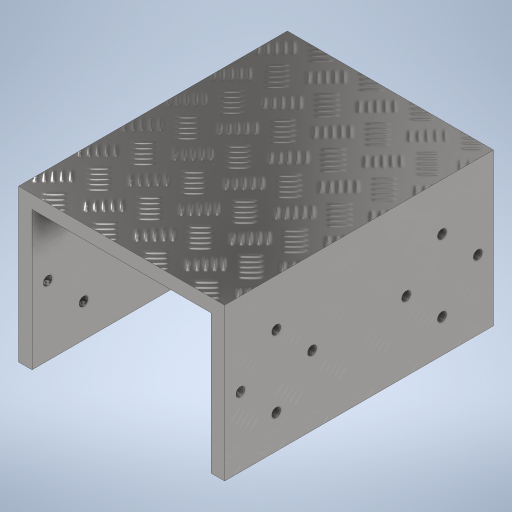
# Autodesk Inventor part: second_junction
Saved by Autodesk Inventor 2024 (Build 280153000, 153)
## iProperties
Created: 2024-02-16
Part Number: second_junction
Material: Generic
Document SubType Name: Modeling
Designer: kamil
Density: 1 g/cm^3
Appearance: Diamond Plate
Author: kamil
Autodesk Inventor part; units mm, degrees
ref_plane "YZ Plane" through (0, 0, 0) normal (1, 0, 0) x (0, 1, 0)
ref_plane "XZ Plane" through (0, 0, 0) normal (0, 1, 0) x (-1, 0, 0)
ref_plane "XY Plane" through (0, 0, 0) normal (0, 0, 1) x (1, 0, 0)
sketch "Sketch1" plane through (0, 0, 0) normal (0, 1, 0) x (-1, 0, 0)
  line L0 (0, 0) -> (46, 0)
  line L1 (46, 0) -> (46, -60)
  line L2 (46, -60) -> (0, -60)
  line L3 (0, -60) -> (0, 0)
  dimension "d0" = 46
  dimension "d1" = 60
  constraints: 8 end point, 2 parallel, 1 horizontal, 1 perpendicular
  measures "d0" distance of L1.end L2.end
  measures "d1" distance of L0.end L1.end
extrude "Extrusion1" add sketch "Sketch1" along normal blind 3
sketch "Sketch2" plane through (0, 0, 0) normal (0, -1, 0) x (1, 0, 0)
  line L0 (-46, -60) -> (-46, 0) projected
  line L1 (-46, 0) -> (0, 0) projected
  line L2 (-46, -60) -> (-43, -60)
  line L3 (-43, -60) -> (-43, 0)
  line L4 (-43, 0) -> (-46, 0)
  line L5 (-46, 0) -> (-46, -60)
  line L6 (0, -60) -> (-46, -60) projected
  line L7 (0, -60) -> (-3, -60)
  line L8 (-3, -60) -> (-3, 0)
  line L9 (-3, 0) -> (0, 0)
  line L10 (0, 0) -> (0, -60)
  dimension "d4" = 3
  dimension "d5" = 3
  dimension "d6" = 60
  constraints: 16 end point, 4 parallel, 2 horizontal, 2 perpendicular, 1 point on line
  measures "d4" distance of L4.end L3.end
  measures "d5" distance of L8.end L9.end
  measures "d6" distance of L7.end L8.end
extrude "Extrusion2" add sketch "Sketch2" along normal blind 31 contours L0 L1 L3 L2 | L8 L1 L10 L6
sketch "Sketch3" plane through (0, 3, 0) normal (1, 0, 0) x (0, 0, -1)
  line L0 (0, -3) -> (0, -34) projected
  line L1 (0, -18.5) -> (11.5, -18.5)
  circle A0 centre (19.5, -18.5) radius 1
  circle A1 centre (11.5, -10.5) radius 1
  circle A2 centre (3.5, -18.5) radius 1
  circle A3 centre (11.5, -26.5) radius 1
  line L2 (60, -3) -> (60, -34) projected
  line L3 (60, -18.5) -> (48.5, -18.5)
  circle A4 centre (40.5, -18.5) radius 1
  circle A5 centre (48.5, -26.5) radius 1
  circle A6 centre (56.5, -18.5) radius 1
  circle A7 centre (48.5, -10.5) radius 1
  dimension "d9" = 11.5
  dimension "d10" = 2
  dimension "d11" = 8
  dimension "d14" = 360
  dimension "d16" = 11.5
  dimension "d17" = 2
  dimension "d18" = 8
  dimension "d21" = 360
  constraints: 8 centre point, 4 end point, 2 midpoint, 1 horizontal, 1 point on line, 18 other
  measures "d9" distance of L1.start L1.end
  measures "d10" diameter of A0
  measures "d11" distance of L1.end A0.centre
  measures "d16" distance of L3.start L3.end
  measures "d17" diameter of A4
  measures "d18" distance of L3.end A4.centre
extrude "Extrusion3" cut sketch "Sketch3" against normal blind 50
body "Solid1"
